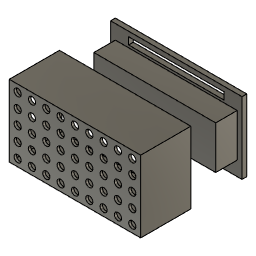
esp82 (Autodesk Fusion 360 design; units mm, degrees)
Autodesk Fusion 360 part; units mm, degrees
note: some values were not read from the file. Set by a fixed rule: which sketch regions a step uses.
sketch "Skizze1" plane through (0, 0, 0) normal (0, 1, 0) x (1, 0, 0)
  line L0 (0, 0) -> (55, 0)
  line L1 (55, 0) -> (55, 30)
  line L2 (55, 30) -> (0, 30)
  line L3 (0, 30) -> (0, 0)
  line L4 (0, 2) -> (56, 2)
  line L5 (56, 2) -> (56, 5)
  line L6 (56, 5) -> (0, 5)
  line L7 (0, 5) -> (0, 2)
  line L8 (0, 2) -> (7.5, 2)
  line L9 (7.5, 2) -> (7.5, 33)
  line L10 (7.5, 33) -> (0, 33)
  line L11 (0, 33) -> (0, 2)
  line L12 (55, 2) -> (47.5, 2)
  line L13 (47.5, 2) -> (47.5, 37)
  line L14 (47.5, 37) -> (55, 37)
  line L15 (55, 37) -> (55, 2)
  line L16 (0, 30) -> (64, 30)
  line L17 (64, 30) -> (64, 28)
  line L18 (64, 28) -> (0, 28)
  line L19 (0, 28) -> (0, 30)
  line L20 (7.5, 28) -> (47.5, 28)
  line L21 (47.5, 28) -> (47.5, 25)
  line L22 (47.5, 25) -> (7.5, 25)
  line L23 (7.5, 25) -> (7.5, 28)
  line L24 (0, 0) -> (2.5, 0)
  line L25 (2.5, 0) -> (2.5, 30)
  line L26 (2.5, 30) -> (0, 30)
  line L27 (0, 30) -> (0, 0)
  line L28 (55, 0) -> (52.5, 0)
  line L29 (52.5, 0) -> (52.5, 30)
  line L30 (52.5, 30) -> (55, 30)
  line L31 (55, 30) -> (55, 0)
  line L32 (-10, 0) -> (65, 0)
  line L33 (65, 0) -> (65, 6)
  line L34 (65, 6) -> (-10, 6)
  line L35 (-10, 6) -> (-10, 0)
  line L36 (-5, 30) -> (70, 30)
  line L37 (70, 30) -> (70, 24)
  line L38 (70, 24) -> (-5, 24)
  line L39 (-5, 24) -> (-5, 30)
  dimension "d1" = 55
  dimension "d2" = 30
  dimension "d3" = 7.5
  dimension "d4" = 7.5
  dimension "d5" = 3
  dimension "d6" = 2.5
  dimension "d7" = 2.5
  constraint horizontal L0
  constraint vertical L1
  constraint horizontal L2
  constraint vertical L3
  constraint coincident L0.start L3.end
  constraint horizontal L4
  constraint vertical L5
  constraint horizontal L6
  constraint vertical L7
  constraint coincident L3 L4.start
  constraint horizontal L8
  constraint vertical L9
  constraint horizontal L10
  constraint vertical L11
  constraint horizontal L12
  constraint vertical L13
  constraint horizontal L14
  constraint vertical L15
  constraint coincident L4 L12.start
  constraint coincident L1 L12.start
  constraint horizontal L16
  constraint vertical L17
  constraint horizontal L18
  constraint vertical L19
  constraint horizontal L20
  constraint vertical L21
  constraint horizontal L22
  constraint vertical L23
  constraint coincident L9 L20.start
  constraint coincident L18 L20.start
  constraint horizontal L24
  constraint vertical L25
  constraint horizontal L26
  constraint vertical L27
  constraint horizontal L28
  constraint vertical L29
  constraint horizontal L30
  constraint vertical L31
  constraint horizontal L32
  constraint vertical L33
  constraint horizontal L34
  constraint vertical L35
  constraint horizontal L36
  constraint vertical L37
  constraint horizontal L38
  constraint vertical L39
  measures "d1" distance of L0.start L0.end
  measures "d2" distance of L0.start L2.end
  measures "d3" distance of L13 L15
  measures "d4" distance of L9.end L10.end
  measures "d5" distance of L20.start L22.end
  measures "d6" distance of L0.start L24.end
  measures "d7" distance of L0.end L28.end
extrude "Extrusion1" add sketch "Skizze1" along normal blind 2 contours L0 L3 L4 L8 L24 L25 L27 L32 | L0 L4 L8 L12 L25 L29 L32 | L3 L4 L6 L7 L8 L11 L25 L27 | L0 L1 L4 L12 L28 L29 L31 L32 | L4 L6 L8 L9 L25 | L3 L6 L11 L25 L27 L34 | L1 L4 L6 L12 L15 L29 L31 | L4 L6 L12 L13 L29 | L4 L6 L9 L13 | L6 L9 L25 L34 | L3 L11 L25 L27 L34 L38 | L1 L6 L15 L29 L31 L34 | L6 L13 L29 L34 | L6 L9 L13 L34 | L9 L25 L34 L38 | L3 L11 L18 L25 L27 L38 | L13 L29 L34 L38 | L1 L15 L29 L31 L34 L38 | L9 L13 L34 L38 | L9 L18 L23 L25 L38 | L2 L3 L11 L16 L18 L19 L25 L26 L27 L36 | L13 L18 L21 L29 L38 | L1 L15 L18 L29 L31 L38 | L9 L13 L22 L38 | L2 L9 L16 L18 L25 L36 | L1 L2 L15 L16 L18 L29 L30 L31 L36 | L2 L13 L16 L18 L29 L36 | L9 L13 L18 L20 L21 L22 L23 | L2 L9 L13 L16 L18 L20 L36 makes body 1
extrude "Extrusion2" cut sketch "Skizze1" along normal blind 15 contours L4 L6 L9 L13 | L9 L13 L18 L20 L21 L22 L23 bodies 1
extrude "Extrusion3" add sketch "Skizze1" against normal blind 9 contours L9 L25 L34 L38 | L13 L29 L34 L38 | L9 L13 L34 L38 bodies 1
extrude "Extrusion4" add 1 faces at (2.5, -3, -12) along direction (-1, 0, 0) blind 0.5 on bodies 1 bodies 1
extrude "Extrusion5" add 1 faces at (52.5, -3, -12) along direction (1, 0, 0) blind 0.5 on bodies 1 bodies 1
sketch "Skizze2" plane through (0, 0, 0) normal (0, -1, 0) x (1, 0, 0)
  line L0 (53, -24) -> (2, -24)
  line L1 (2, -24) -> (2, -6)
  line L2 (2, -6) -> (53, -6)
  line L3 (53, -6) -> (53, -24)
  line L4 (0, -30) -> (55, -30)
  line L5 (55, -30) -> (55, 0)
  line L6 (55, 0) -> (0, 0)
  line L7 (0, 0) -> (0, -30)
  line L8 (7.5, -28) -> (7.5, -25)
  line L9 (7.5, -25) -> (47.5, -25)
  line L10 (47.5, -25) -> (47.5, -28)
  line L11 (47.5, -28) -> (7.5, -28)
  line L12 (7.5, -5) -> (7.5, -2)
  line L13 (7.5, -2) -> (47.5, -2)
  line L14 (47.5, -2) -> (47.5, -5)
  line L15 (47.5, -5) -> (7.5, -5)
  line L16 (1, -29) -> (54, -29)
  line L17 (54, -29) -> (54, -1)
  line L18 (54, -1) -> (1, -1)
  line L19 (1, -1) -> (1, -29)
  dimension "d18" = -1
extrude "Extrusion6" add sketch "Skizze2" along normal blind 20 separate body contours L4 L5 L6 L7 makes body 2
sketch "Skizze3" plane through (0, -20, 0) normal (0, -1, 0) x (1, 0, 0)
  line L0 (1, -29) -> (1, -1)
  line L1 (1, -1) -> (54, -1)
  line L2 (54, -1) -> (54, -29)
  line L3 (54, -29) -> (1, -29)
  line L4 (0, 0) -> (0, -30)
  line L5 (0, -30) -> (55, -30)
  line L6 (55, -30) -> (55, 0)
  line L7 (55, 0) -> (0, 0)
  line L8 (0, 0) -> (55, 0)
  line L9 (55, 0) -> (55, -30)
  line L10 (55, -30) -> (0, -30)
  line L11 (0, -30) -> (0, 0)
  constraint horizontal L8
  constraint vertical L9
  constraint horizontal L10
  constraint vertical L11
  constraint coincident L5.end L6.start
  constraint coincident L4.start L7.end
extrude "Extrusion7" add sketch "Skizze3" along normal blind 1 contours L0 L1 L2 L3 | L4 L5 L6 L7 L8 L9 L10 L11 bodies 2
sketch "Skizze4" plane through (0, 0, 0) normal (-1, 0, 0) x (0, -1, 0)
  line L0 (0, 0) -> (0, -30)
  line L1 (0, -30) -> (21, -30)
  line L2 (21, -30) -> (21, 0)
  line L3 (21, 0) -> (0, 0)
  line L4 (10, -10) -> (16, -10)
  line L5 (16, -10) -> (16, -20)
  line L6 (16, -20) -> (10, -20)
  line L7 (10, -20) -> (10, -10)
  constraint horizontal L4
  constraint vertical L5
  constraint horizontal L6
  constraint vertical L7
extrude "Extrusion8" cut sketch "Skizze4" against normal blind 4 contours L4 L5 L6 L7 bodies 2
sketch "Skizze5" plane through (0, -21, 0) normal (0, -1, 0) x (1, 0, 0)
  line L0 (0, -30) -> (55, -30)
  line L1 (55, -30) -> (55, 0)
  line L2 (55, 0) -> (0, 0)
  line L3 (0, 0) -> (0, -30)
  line L4 (0, 0) -> (55, -30)
  line L5 (55, 0) -> (0, -30)
  circle A0 centre (27.5, -15) radius 1.5
  circle A1 centre (3.5, -27) radius 1.5
  circle A2 centre (9.5, -27) radius 1.5
  circle A3 centre (15.5, -27) radius 1.5
  circle A4 centre (21.5, -27) radius 1.5
  circle A5 centre (27.5, -27) radius 1.5
  circle A6 centre (33.5, -27) radius 1.5
  circle A7 centre (39.5, -27) radius 1.5
  circle A8 centre (45.5, -27) radius 1.5
  circle A9 centre (51.5, -27) radius 1.5
  circle A10 centre (3.5, -21) radius 1.5
  circle A11 centre (9.5, -21) radius 1.5
  circle A12 centre (15.5, -21) radius 1.5
  circle A13 centre (21.5, -21) radius 1.5
  circle A14 centre (27.5, -21) radius 1.5
  circle A15 centre (33.5, -21) radius 1.5
  circle A16 centre (39.5, -21) radius 1.5
  circle A17 centre (45.5, -21) radius 1.5
  circle A18 centre (51.5, -21) radius 1.5
  circle A19 centre (3.5, -15) radius 1.5
  circle A20 centre (9.5, -15) radius 1.5
  circle A21 centre (15.5, -15) radius 1.5
  circle A22 centre (21.5, -15) radius 1.5
  circle A23 centre (33.5, -15) radius 1.5
  circle A24 centre (39.5, -15) radius 1.5
  circle A25 centre (45.5, -15) radius 1.5
  circle A26 centre (51.5, -15) radius 1.5
  circle A27 centre (3.5, -9) radius 1.5
  circle A28 centre (9.5, -9) radius 1.5
  circle A29 centre (15.5, -9) radius 1.5
  circle A30 centre (21.5, -9) radius 1.5
  circle A31 centre (27.5, -9) radius 1.5
  circle A32 centre (33.5, -9) radius 1.5
  circle A33 centre (39.5, -9) radius 1.5
  circle A34 centre (45.5, -9) radius 1.5
  circle A35 centre (51.5, -9) radius 1.5
  circle A36 centre (3.5, -3) radius 1.5
  circle A37 centre (9.5, -3) radius 1.5
  circle A38 centre (15.5, -3) radius 1.5
  circle A39 centre (21.5, -3) radius 1.5
  circle A40 centre (27.5, -3) radius 1.5
  circle A41 centre (33.5, -3) radius 1.5
  circle A42 centre (39.5, -3) radius 1.5
  circle A43 centre (45.5, -3) radius 1.5
  circle A44 centre (51.5, -3) radius 1.5
  dimension "d25" = 3
  dimension "d28" = 24
  dimension "d29" = 12
  constraint coincident L2.end L3.start
  constraint coincident L0.end L1.start
  constraint coincident L1.end L2.start
  constraint coincident L0.start L3.end
  constraint midpoint L4 A0.centre
  measures "d25" diameter of A0
extrude "Extrusion9" cut sketch "Skizze5" against normal blind 4 contours L5 A1 | L5 A1 | L4 A9 | L4 A9 | L4 A36 | L4 A36 | L5 A44 | L5 A44 | L5 A12 | L5 A12 | L4 A16 | L4 A16 | L4 A29 | L4 A29 | L5 A33 | L5 A33 | L4 L5 A0 | L4 L5 A0 | L4 L5 A0 | L4 L5 A0 | A2 | A3 | A4 | A5 | A6 | A7 | A8 | A10 | A11 | A13 | A14 | A15 | A17 | A18 | A19 | A20 | A21 | A22 | A23 | A24 | A25 | A26 | A27 | A28 | A30 | A31 | A32 | A34 | A35 | A37 | A38 | A39 | A40 | A41 | A42 | A43 bodies 2
copy_body "Körper->Berechn1" bodies 1 removing the originals makes body 3 in component "Component"
copy_body "Körper->Berechn2" bodies 2 removing the originals makes body 4 in component "Component'"
component "Component" placed x (1, 0, 0) y (0, 1, 0) z (0, 0, 1) at (0, 0, 0)
component "Component'" placed x (1, 0, 0) y (0, 1, 0) z (0, 0, 1) at (0, 0, 0)
